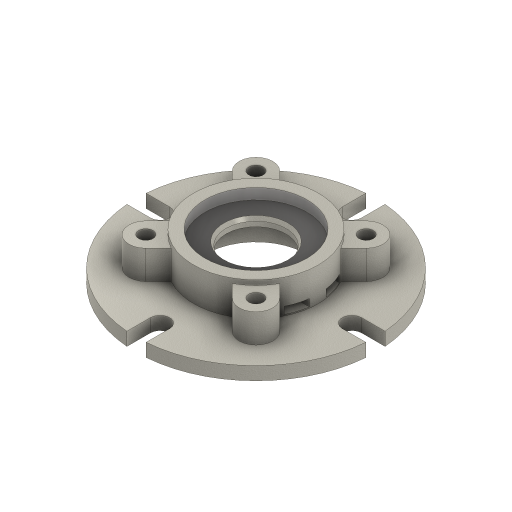
# Autodesk Inventor part: Part038. Flat stand
Saved by Autodesk Inventor 2023.2 (Build 272271030, 271C)
## iProperties
Created: 2023-11-22
Part Number: Part038. Flat stand
Material: Steel, Carbon
Document SubType Name: Modeling
Designer: User
Mass: 3257.14 g
Surface Area: 941.552 cm^2
Volume: 414.923 cm^3
Density: 7.85 g/cm^3
Appearance: Steel - Cast
Author: User
Autodesk Inventor part; units mm, degrees
ref_plane "YZ Plane" through (0, 0, 0) normal (1, 0, 0) x (0, 1, 0)
ref_plane "XZ Plane" through (0, 0, 0) normal (0, 1, 0) x (-1, 0, 0)
ref_plane "XY Plane" through (0, 0, 0) normal (0, 0, 1) x (1, 0, 0)
sketch "Sketch1" plane through (0, 0, 0) normal (0, 0, 1) x (1, 0, 0)
  line L0 (0, 0) -> (0, 39)
  line L1 (42, 0) -> (42, 25.5)
  line L2 (42, 25.5) -> (36, 25.5)
  line L3 (36, 25.5) -> (36, 23)
  line L4 (36, 23) -> (25, 23)
  line L5 (25, 23) -> (25, 27)
  line L6 (25, 27) -> (26.7321, 30)
  line L7 (26.7321, 30) -> (42.5, 30)
  line L8 (42.5, 30) -> (42.5, 39)
  line L9 (42.5, 39) -> (52, 39)
  line L10 (52, 39) -> (52, 11)
  line L11 (52, 11) -> (100, 11)
  line L12 (100, 11) -> (100, 0)
  line L13 (100, 0) -> (42, 0)
  dimension "d0" = 39
  dimension "d1" = 200
  dimension "d2" = 84
  dimension "d3" = 85
  dimension "d4" = 11
  dimension "d5" = 50
  dimension "d6" = 72
  dimension "d7" = 23
  dimension "d8" = 30
  dimension "d9" = 30
  dimension "d10" = 25.5
  dimension "d11" = 104
  dimension "d12" = 3
  constraints: 28 end point, 10 perpendicular, 2 point on line, 2 vertical, 1 parallel
  measures "d0" distance of L0.start L0.end
  measures "d1" diameter of L12 L0
  measures "d2" diameter of L1 L0
  measures "d3" diameter of L8 L0
  measures "d4" distance between parallel lines of L13 L11
  measures "d5" diameter of L5 L0
  measures "d6" diameter of L3 L0
  measures "d7" distance between parallel lines of L13 L4
  measures "d8" angle of L6 L5
  measures "d9" distance between parallel lines of L13 L7
  measures "d10" distance between parallel lines of L13 L2
  measures "d11" diameter of L10 L0
  measures "d12" vertical distance of L5.end L6.end
revolve "Revolution1" add sketch "Sketch1" angle 360 about axis through (0, 0, 0) along (0, 1, 0)
sketch "Sketch2" plane through (0, 0, 0) normal (1, 0, 0) x (0, 1, 0)
  line L0 (18, 23) -> (12, 23)
  line L1 (12, 23) -> (12, 7)
  line L2 (12, 7) -> (18, 7)
  line L3 (18, 7) -> (18, 23)
  line L4 (0, -42) -> (0, 42) projected
  point P0 (0, 0)
  point P1 (0, 0)
  dimension "d14" = 12
  dimension "d15" = 6
  dimension "d16" = 16
  dimension "d17" = 7
  constraints: 8 end point, 2 parallel, 1 horizontal, 1 midpoint, 1 perpendicular
  measures "d14" distance between parallel lines of L4 L1
  measures "d15" distance between parallel lines of L1 L3
  measures "d16" distance between parallel lines of L0 L2
  measures "d17" distance from line of point (0, 0) L2
extrude "Extrusion1" cut sketch "Sketch2" along normal through all both and the other way through all
mirror "Mirror1" about plane through (0, 0, 0) normal (0, 0, 1) of "Extrusion1"
sketch "Sketch3" plane through (0, 11, 0) normal (0, 1, 0) x (1, 0, 0)
  circle A0 centre (0, 0) radius 52 projected
  circle A1 centre (0, 0) radius 100 projected
  line L0 (99.6795, 8) -> (80, 8)
  arc A2 (80, 8) -> (80, -8) centre (80, 0) ccw
  line L1 (80, -8) -> (99.6795, -8)
  arc A3 (99.6795, -8) -> (99.6795, 8) centre (0, 0) ccw
  dimension "d20" = 8
  dimension "d21" = 80
  constraints: 6 point on circle, 4 end point, 2 centre point, 2 tangent, 1 horizontal, 1 horizontal alignment, 1 parallel
  measures "d20" radius of A2
  measures "d21" distance of A0.centre A2.centre
extrude "Extrusion2" cut sketch "Sketch3" against normal through all contours A1 L1 A2 L0 picked at (86.6667, 0)
sketch "Sketch4" plane through (80, 11, -8) normal (0, 1, 0) x (1, 0, 0)
  circle A0 centre (-80, -8) radius 52 projected
  line L0 (-80, -8) -> (-34.0381, 37.9619) construction
  line L1 (-80, -8) -> (-15, -8) construction
  line L2 (-54.4876, 37.3114) -> (-43.9376, 47.8614)
  arc A1 (-24.1386, 28.0624) -> (-43.9376, 47.8614) centre (-34.0381, 37.9619) ccw
  line L3 (-24.1386, 28.0624) -> (-34.6886, 17.5124)
  dimension "d24" = 65
  dimension "d25" = 45
  dimension "d26" = 14
  constraints: 8 end point, 4 point on circle, 2 parallel, 2 tangent, 1 centre point, 1 coincident, 1 equal length, 1 horizontal
  measures "d24" distance of L0.start L0.end
  measures "d25" angle of L1 L0
  measures "d26" radius of A1
extrude "Extrusion3" add sketch "Sketch4" along normal blind 24 contours A0 L2 A1 L3
sketch "Sketch5" plane through (80, 35, -8) normal (0, 1, 0) x (1, 0, 0)
  arc A0 (-24.1386, 28.0624) -> (-43.9376, 47.8614) centre (-34.0381, 37.9619) ccw projected
  point P0 (-80, -8)
  constraints: 1 coincident
hole "Hole1" at (45.9619, 35, -45.9619) direction (0, -1, 0) diameter 12 end through all
pattern_circular "Circular Pattern1" count 4 over 360 about axis through (0, 5.5, 0) along (0, 1, 0) of "Extrusion2", "Extrusion3", "Hole1"
body "Solid1"
